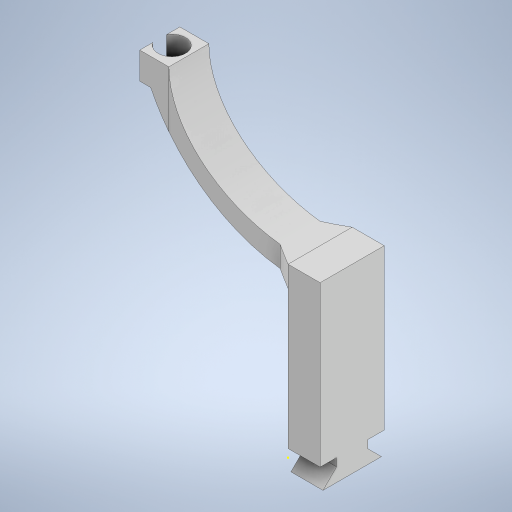
# Autodesk Inventor part: Pasteur_holder_V2
Saved by Autodesk Inventor 2024 (Build 280153000, 153)
## iProperties
Created: 2020-11-04
Part Number: Pasteur_holder_V2
Material: Generic
Document SubType Name: Modeling
Designer: Allesfresser
Density: 1 g/cm^3
Appearance: Default
Author: Allesfresser
Autodesk Inventor part; units mm, degrees
ref_plane "YZ Plane" through (0, 0, 0) normal (1, 0, 0) x (0, 1, 0)
ref_plane "XZ Plane" through (0, 0, 0) normal (0, 1, 0) x (-1, 0, 0)
ref_plane "XY Plane" through (0, 0, 0) normal (0, 0, 1) x (1, 0, 0)
sketch "Sketch1" plane through (0, 0, 0) normal (1, 0, 0) x (0, 1, 0)
  line L0 (0, 0) -> (0, 3.9)
  line L1 (0, 0) -> (0, -3.9)
  line L2 (0, 3.9) -> (-3.3941, 7.2941)
  line L3 (0, 3.9) -> (4.8, 3.9) construction
  line L4 (0, -3.9) -> (-3.3941, -7.2941)
  line L5 (0, -3.9) -> (4.8, -3.9) construction
  line L6 (-3.3941, -7.2941) -> (-3.3941, 7.2941)
  dimension "d0" = 3.9
  dimension "d1" = 3.9
  dimension "d2" = 4.8
  dimension "d3" = 135
  dimension "d4" = 4.8
  dimension "d5" = 135
  constraints: 14 end point, 2 equal length, 2 horizontal, 2 vertical
  measures "d0" distance of L0.start L0.end
  measures "d1" distance of L0.start L1.end
  measures "d2" distance of L0.end L2.end
  measures "d3" angle of L3 L2
  measures "d4" distance of L1.end L4.end
  measures "d5" angle of L4 L5
extrude "Extrusion1" add sketch "Sketch1" along normal blind 8
sketch "Sketch2" plane through (0, 0, 3.9) normal (0, 1, 0) x (1, 0, 0)
  line L0 (0, -3.3941) -> (0, 11.1941) projected
  line L1 (0, -0.0082) -> (8, -0.0082)
  line L2 (8, -0.0082) -> (8, 7.7918)
  line L3 (8, 7.7918) -> (0, 7.7918)
  line L4 (0, 7.7918) -> (0, -0.0082)
  point P0 (0, 3.9)
  dimension "d8" = 8
  dimension "d9" = 7.8
  constraints: 8 end point, 2 parallel, 1 horizontal, 1 perpendicular, 1 point on line
  measures "d8" distance of L3.end L2.end
  measures "d9" distance of L2.end L1.end
extrude "Extrusion2" add sketch "Sketch2" along normal blind 2
sketch "Sketch3" plane through (0, 2, 3.9) normal (0, 1, 0) x (1, 0, 0)
  line L0 (8, -4.1082) -> (0, -4.1082)
  line L1 (0, -4.1082) -> (0, 11.8918)
  line L2 (0, 11.8918) -> (8, 11.8918)
  line L3 (8, 11.8918) -> (8, -4.1082)
  line L4 (8, -4.1082) -> (0, 11.8918) construction
  line L5 (0, -4.1082) -> (8, 11.8918) construction
  line L6 (8, 7.7918) -> (0, 7.7918) projected
  point P0 (0, 3.9)
  point P1 (4, 3.8918)
  dimension "d12" = 8
  dimension "d13" = 16
  dimension "d14" = 3.9
  dimension "d15" = 4
  constraints: 12 end point, 2 midpoint, 2 parallel, 1 horizontal, 1 perpendicular
  measures "d12" distance of L1.end L2.end
  measures "d13" distance of L0.end L1.end
  measures "d14" distance from line of L6 point (4, 3.892)
  measures "d15" distance of point (0, 3.9) point (4, 3.892)
extrude "Extrusion3" add sketch "Sketch3" along normal blind 64.606
sketch "Sketch4" plane through (0, 0, 0) normal (-1, 0, 0) x (0, 0, 1)
  line L0 (-7.9918, 2) -> (-7.9918, 66.606) projected
  line L1 (8.0082, 2) -> (8.0082, 66.606) projected
  line L2 (-7.9918, 66.606) -> (8.0082, 66.606)
  line L3 (8.0082, 66.606) -> (8.0082, 36.606)
  line L4 (8.0082, 36.606) -> (-7.9918, 36.606)
  line L5 (-7.9918, 36.606) -> (-7.9918, 66.606)
  point P0 (0, 0)
  point P1 (8.0082, 66.606)
  point P2 (-7.9918, 36.606)
  dimension "d18" = 30
  constraints: 8 end point, 2 parallel, 1 horizontal, 1 perpendicular, 1 point on line
  measures "d18" distance of L2.end L3.end
extrude "Extrusion4" add sketch "Sketch4" along normal blind 40
sketch "Sketch5" plane through (0, 66.606, 3.9) normal (0, 1, 0) x (1, 0, 0)
  circle A0 centre (-37, 3.8918) radius 3.45
  line L0 (-40, -4.1082) -> (-40, 11.8918) projected
  line L1 (8, 11.8918) -> (-40, 11.8918) projected
  point P0 (0, 3.9)
  point P1 (-40, 5.5955)
  point P2 (-40, 2.1882)
  dimension "d21" = 6.9
  dimension "d22" = 3
  dimension "d53" = 8
  constraints: 1 centre point
  measures "d21" diameter of A0
  measures "d22" distance from line of A0.centre L0
  measures "d53" distance from line of L1 A0.centre
sketch "Sketch6" plane through (0, 2, 8.0082) normal (0, 0, 1) x (1, 0, 0)
  point P0 (0, -2)
sketch "Sketch7" plane through (0, 2, 8.0082) normal (0, 0, 1) x (1, 0, 0)
  point P0 (0, -2)
sketch "Sketch10" plane through (0, 2, 8.0082) normal (0, 0, 1) x (1, 0, 0)
  ellipse E0 centre (0, 64.6805) end of major axis (0, 39.8349) minor radius 32.7521
  line L0 (8, 64.606) -> (-40, 64.606) projected
  line L1 (0, 39.8349) -> (8, 39.8349)
  line L2 (8, 39.8349) -> (8, 64.606)
  line L3 (8, 64.606) -> (0, 64.606)
  line L4 (0, 64.606) -> (0, 39.8349)
  point P0 (0, -2)
  point P1 (8, 40.5875)
  constraints: 8 end point, 2 parallel, 1 horizontal, 1 perpendicular, 3 other
extrude "Extrusion8" cut sketch "Sketch10" against normal through all
sketch "Sketch13" plane through (0, 36.606, -7.9918) normal (0, -1, 0) x (1, 0, 0)
  circle A0 centre (-37.1694, 8) radius 4.375
  line L0 (0, 16) -> (-40, 16) projected
  point P0 (0, 7.9918)
  dimension "d37" = 8.75
  dimension "d46" = 8
  constraints: 1 centre point
  measures "d37" diameter of A0
  measures "d46" distance from line of A0.centre L0
extrude "Extrusion9" cut sketch "Sketch13" against normal blind 24
extrude "Extrusion10" cut sketch "Sketch5" against normal blind 24
sketch "Sketch14" plane through (8, 2, -7.9918) normal (0, 0, -1) x (-1, 0, 0)
  line L0 (48, 34.606) -> (40.7944, 34.606) projected
  line L1 (45.2609, 34.606) -> (48, 34.606)
  line L2 (48, 34.606) -> (48, 57.8825)
  line L3 (48, 57.8825) -> (45.2609, 57.8825)
  line L4 (45.2609, 57.8825) -> (45.2609, 34.606)
  point P0 (8, -2)
  constraints: 8 end point, 2 parallel, 1 horizontal, 1 perpendicular, 1 point on line
extrude "Extrusion11" cut sketch "Sketch14" against normal blind 24
sketch "Sketch15" plane through (0, 2, 8.0082) normal (0, 0, 1) x (1, 0, 0)
  line L0 (-37.2609, 57.8825) -> (-37.2609, 34.606) projected
  line L1 (0, 34.606) -> (-37.2609, 34.606) projected
  arc A0 (-37.2609, 57.8825) -> (0, 34.606) centre (-0.1523, 75.824) ccw
  point P0 (0, -2)
  point P1 (-0.3046, 34.606)
  constraints: 2 point on circle, 1 centre point
extrude "Extrusion12" cut sketch "Sketch15" against normal through all
sketch "Sketch16" plane through (0, 66.606, 3.9) normal (0, 1, 0) x (1, 0, 0)
  line L0 (-40, 5.5955) -> (-40, 11.8918) projected
  line L1 (-32.752, 11.8918) -> (-40, 11.8918) projected
  line L2 (-32.752, -4.1082) -> (-32.752, 11.8918) projected
  line L3 (-40, 11.8918) -> (-32.752, 11.8918)
  line L4 (-32.752, 11.8918) -> (-32.752, 8.8918)
  line L5 (-32.752, 8.8918) -> (-40, 8.8918)
  line L6 (-40, 8.8918) -> (-40, 11.8918)
  line L7 (0, 11.8918) -> (0, 7.7918) projected
  line L8 (0, 11.8918) -> (-5, 11.8918)
  line L9 (-5, 11.8918) -> (-5, 8.8755)
  line L10 (-5, 8.8755) -> (0, 8.8755)
  line L11 (0, 8.8755) -> (0, 11.8918)
  line L12 (-5, 8.8755) -> (-32.752, 8.8755)
  line L13 (-32.752, 8.8755) -> (-32.752, 11.8918)
  line L14 (-32.752, 11.8918) -> (-5, 11.8918)
  line L15 (-5, 11.8918) -> (-5, 8.8755)
  line L16 (0, 11.8918) -> (-5, 8.8755)
  line L17 (0, 3.8918) -> (-40, 3.8918)
  line L18 (-40, 2.1882) -> (-40, -4.1082)
  line L19 (-32.752, -4.1082) -> (-40, -4.1082)
  line L20 (-32.752, 11.8918) -> (-32.752, -4.1082)
  line L21 (-40, -4.1082) -> (-32.752, -4.1082)
  line L22 (-32.752, -4.1082) -> (-32.752, -1.1082)
  line L23 (-32.752, -1.1082) -> (-40, -1.1082)
  line L24 (-40, -1.1082) -> (-40, -4.1082)
  line L25 (0, -4.1082) -> (0, -0.0082)
  line L26 (0, -4.1082) -> (-5, -4.1082)
  line L27 (-5, -4.1082) -> (-5, -1.0918)
  line L28 (-5, -1.0918) -> (0, -1.0918)
  line L29 (0, -1.0918) -> (0, -4.1082)
  line L30 (-5, -1.0918) -> (-32.752, -1.0918)
  line L31 (-32.752, -1.0918) -> (-32.752, -4.1082)
  line L32 (-32.752, -4.1082) -> (-5, -4.1082)
  line L33 (-5, -4.1082) -> (-5, -1.0918)
  line L34 (0, -4.1082) -> (-5, -1.0918)
  point P0 (0, -1.0918)
  dimension "d48" = 3
  dimension "d49" = 5
  dimension "d52" = 8
  constraints: 62 end point, 14 symmetric about line, 6 parallel, 4 horizontal, 3 perpendicular, 2 point on line
  measures "d48" distance of L3.end L4.end
  measures "d49" distance of L10.end L9.end
  measures "d52" distance between parallel lines of L14 L17
extrude "Extrusion13" cut sketch "Sketch16" against normal through all contours L30 L27 L32 L2 | L0 L1 L2 L5 | L2 L14 L9 L12 | L8 L16 L9 | L2 L19 L18 L23 | L34 L26 L27
body "Solid1"
